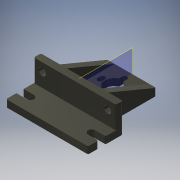
# Autodesk Inventor part: Z Nut Braket 1.0
Saved by Autodesk Inventor 2016 (Build 200138000, 138)
## iProperties
Created: 2017-04-04
Part Number: Z Nut Braket 1.0
Material: PC/ABS Plastic
Document SubType Name: Modeling
Designer: Scott
Density: 0.357273 g/cm^3
Appearance: Gunmetal
Author: Scott
Autodesk Inventor part; units mm, degrees
ref_plane "YZ Plane" through (0, 0, 0) normal (1, 0, 0) x (0, 1, 0)
ref_plane "XZ Plane" through (0, 0, 0) normal (0, 1, 0) x (-1, 0, 0)
sketch "Sketch1" plane through (0, 0, 0) normal (0, 0, 1) x (1, 0, 0)
  line L0 (9.5028, 23.3821) -> (9.5028, -12.6179)
  line L1 (14.5028, 23.3821) -> (14.5028, -12.6179)
  line L2 (26.5028, -12.6179) -> (26.5028, -37.6179)
  line L3 (-32.4972, -17.6179) -> (26.5028, -17.6179)
  line L4 (-32.4972, -12.6179) -> (-20.4972, -12.6179)
  line L5 (-15.4972, -12.6179) -> (9.5028, -12.6179)
  line L6 (14.5028, -12.6179) -> (26.5028, -12.6179)
  line L7 (-20.4972, 23.3821) -> (14.5028, 23.3821)
  line L8 (-15.4972, 23.3821) -> (-15.4972, -12.6179)
  line L9 (-20.4972, 23.3821) -> (-20.4972, -12.6179)
  line L10 (-32.4972, -37.6179) -> (26.5028, -37.6179)
  line L11 (-32.4972, -12.6179) -> (-32.4972, -37.6179)
  line L12 (-2.9972, 1.3821) -> (-2.9972, 17.3821) construction
  line L13 (5.0028, 9.3821) -> (-10.9972, 9.3821) construction
  circle A0 centre (-2.9972, 9.3821) radius 8 construction
  line L14 (-2.9972, 10.3821) -> (-2.9972, 8.3821) construction
  line L15 (-8.4972, 10.3821) -> (-8.4972, 8.3821)
  line L16 (2.5028, 8.3821) -> (2.5028, 10.3821)
  line L17 (-2.9972, 2.3821) -> (-2.9972, 0.3821) construction
  line L18 (-4.7472, 2.3821) -> (-4.7472, 0.3821)
  line L19 (-1.2472, 0.3821) -> (-1.2472, 2.3821)
  arc A1 (-4.7472, 0.3821) -> (-1.2472, 0.3821) centre (-2.9972, 0.3821) ccw
  line L20 (-10.9972, 10.3821) -> (-10.9972, 8.3821) construction
  line L21 (-12.7472, 10.3821) -> (-12.7472, 8.3821)
  line L22 (-9.2472, 8.3821) -> (-9.2472, 10.3821)
  arc A2 (-9.2472, 10.3821) -> (-12.7472, 10.3821) centre (-10.9972, 10.3821) ccw
  arc A3 (-12.7472, 8.3821) -> (-9.2472, 8.3821) centre (-10.9972, 8.3821) ccw
  line L23 (5.0028, 10.3821) -> (5.0028, 8.3821) construction
  line L24 (3.2528, 10.3821) -> (3.2528, 8.3821)
  line L25 (6.7528, 8.3821) -> (6.7528, 10.3821)
  arc A4 (6.7528, 10.3821) -> (3.2528, 10.3821) centre (5.0028, 10.3821) ccw
  arc A5 (3.2528, 8.3821) -> (6.7528, 8.3821) centre (5.0028, 8.3821) ccw
  line L26 (-2.9972, 18.3821) -> (-2.9972, 16.3821) construction
  line L27 (-1.2472, 18.3821) -> (-1.2472, 16.3821)
  line L28 (-4.7472, 16.3821) -> (-4.7472, 18.3821)
  arc A6 (-1.2472, 18.3821) -> (-4.7472, 18.3821) centre (-2.9972, 18.3821) ccw
  arc A7 (-1.2472, 2.3821) -> (-1.4087, 3.1165) centre (-2.9972, 2.3821) ccw
  arc A8 (-4.5856, 3.1165) -> (-4.7472, 2.3821) centre (-2.9972, 2.3821) ccw
  arc A9 (-8.4972, 8.3821) -> (-4.5856, 3.1165) centre (-2.9972, 8.3821) ccw
  arc A10 (-1.4087, 3.1165) -> (2.5028, 8.3821) centre (-2.9972, 8.3821) ccw
  arc A11 (-4.7472, 16.3821) -> (-4.5856, 15.6478) centre (-2.9972, 16.3821) ccw
  arc A12 (-1.4087, 15.6478) -> (-1.2472, 16.3821) centre (-2.9972, 16.3821) ccw
  arc A13 (2.5028, 10.3821) -> (-1.4087, 15.6478) centre (-2.9972, 10.3821) ccw
  arc A14 (-4.5856, 15.6478) -> (-8.4972, 10.3821) centre (-2.9972, 10.3821) ccw
  point P0 (0, 0)
  point P1 (14.5028, 29.202)
  point P2 (-20.4972, 29.202)
  dimension "d51" = 16
  dimension "d52" = 5
  dimension "d53" = 5
  dimension "d54" = 25
  dimension "d55" = 5
  dimension "d56" = 20
  dimension "d58" = 27
  dimension "d59" = 14
  dimension "d60" = 12
  dimension "d61" = 12
  dimension "d64" = 12.5
  dimension "d66" = 2
  dimension "d67" = 3.5
  dimension "d68" = 2
  dimension "d69" = 3.5
  dimension "d70" = 2
  dimension "d71" = 3.5
  dimension "d72" = 2
  dimension "d73" = 3.5
  dimension "d74" = 2
  constraints: 68 end point, 33 point on circle, 22 tangent, 15 centre point, 13 parallel, 8 point on line, 7 midpoint, 5 vertical, 3 coincident, 2 collinear, 2 horizontal
  measures "d51" diameter of A0
  measures "d52" distance between parallel lines of L9 L8
  measures "d53" distance between parallel lines of L1 L0
  measures "d54" distance between parallel lines of L8 L0
  measures "d55" distance between parallel lines of L4 L3
  measures "d56" distance between parallel lines of L10 L3
  measures "d58" distance between parallel lines of L13 L3
  measures "d59" distance between parallel lines of L7 L13
  measures "d60" distance between parallel lines of L1 L2
  measures "d61" distance between parallel lines of L11 L9
  measures "d64" distance between parallel lines of L0 L12
  measures "d66" distance of L15.start L15.end
  measures "d67" diameter of A1
  measures "d68" distance of L18.start L18.end
  measures "d69" diameter of A3
  measures "d70" distance of L21.start L21.end
  measures "d71" diameter of A5
  measures "d72" distance of L25.start L25.end
  measures "d73" distance between parallel lines of L28 L27
  measures "d74" distance of L28.start L28.end
extrude "Extrusion1" add sketch "Sketch1" along normal blind 5
sketch "Sketch2" plane through (0, 0, 5) normal (0, 0, 1) x (1, 0, 0)
  line L0 (26.5028, -37.6179) -> (26.5028, -12.6179) projected
  line L1 (-32.4972, -12.6179) -> (26.5028, -12.6179)
  line L2 (26.5028, -12.6179) -> (26.5028, -17.6179)
  line L3 (26.5028, -17.6179) -> (-32.4972, -17.6179)
  line L4 (-32.4972, -17.6179) -> (-32.4972, -12.6179)
  line L5 (-32.4972, -12.6179) -> (-32.4972, -37.6179) projected
  line L6 (26.5028, -12.6179) -> (14.5028, -12.6179) projected
  point P0 (0, 0)
  dimension "d30" = 5
  constraints: 8 end point, 2 collinear, 2 parallel, 1 horizontal, 1 perpendicular, 1 point on line
  measures "d30" distance between parallel lines of L1 L3
extrude "Extrusion2" add sketch "Sketch2" along normal blind 16
sketch "Sketch3" plane through (14.5028, -12.6179, 0) normal (1, 0, 0) x (0, 0, -1)
  line L0 (0, 0) -> (-21, 0) projected
  line L1 (-5, 0) -> (-5, 36) projected
  line L2 (-21, 0) -> (-5, 0)
  line L3 (-5, 36) -> (-20, 0)
  point P0 (0, 12.6179)
  point P1 (-5, 31)
  dimension "d77" = 15
  constraints: 4 end point, 1 perpendicular, 1 point on line
  measures "d77" distance from line of L1 L3.end
extrude "Extrusion3" add sketch "Sketch3" against normal blind 5
sketch "Sketch4" plane through (14.5028, -12.6179, 0) normal (0, 1, 0) x (1, 0, 0)
  circle A0 centre (6, -15) radius 2.6
  line L0 (12, 0) -> (12, -21) projected
  line L1 (12, -21) -> (-47, -21) projected
  point P0 (-14.5028, 0)
  point P1 (0, -25)
  dimension "d36" = 5.2
  dimension "d37" = 6
  dimension "d38" = 6
  constraints: 1 centre point, 1 other
  measures "d36" diameter of A0
  measures "d37" distance from line of L0 A0.centre
extrude "Extrusion4" cut sketch "Sketch4" against normal through all
sketch "Sketch5" plane through (0, 0, 5) normal (0, 0, 1) x (1, 0, 0)
  arc A0 (19.0028, -25.0179) -> (19.0028, -30.2179) centre (19.0028, -27.6179) ccw
  line L0 (26.5028, -37.6179) -> (26.5028, -17.6179) projected
  line L1 (-32.4972, -37.6179) -> (26.5028, -37.6179) projected
  line L2 (19.0028, -25.0179) -> (26.5028, -25.0179)
  line L3 (19.0028, -30.2179) -> (26.5028, -30.2179)
  line L4 (26.5028, -37.6179) -> (26.5028, -12.6179) projected
  line L5 (26.5028, -25.0179) -> (26.5028, -30.2179)
  point P0 (0, 0)
  point P1 (-34.4972, -33.6179)
  point P2 (17.5028, -33.6179)
  dimension "d41" = 7.5
  dimension "d42" = 10
  dimension "d43" = 5.2
  constraints: 6 end point, 2 point on circle, 2 point on line, 2 tangent, 1 centre point, 1 collinear, 1 horizontal, 1 perpendicular, 1 other
  measures "d41" distance from line of L0 A0.centre
  measures "d43" diameter of A0
extrude "Extrusion5" cut sketch "Sketch5" against normal blind 5
fillet "Fillet1" radius 1 5 edges at (-32.4972, -12.6179, 10.5) (-32.4972, -17.6179, 13) (26.5028, -30.2179, 2.5) (26.5028, -25.0179, 2.5) (26.5028, -17.6179, 13)
ref_plane "Work Plane2" through (-2.9972, 0.3821, 0) normal (1, 0, 0) x (0, 0, 1)
mirror "Mirror2" about plane through (-2.9972, 0.3821, 0) normal (1, 0, 0) of "Extrusion5", "Extrusion4", "Extrusion3"
fillet "Fillet2" radius 1 8 edges at (14.5028, 23.3821, 2.5) (-20.4972, 23.3821, 2.5) (26.5028, -37.6179, 2.5) (-32.4972, -37.6179, 2.5) (-1.4087, 3.1165, 2.5) (-4.5856, 3.1165, 2.5) (-1.4087, 15.6478, 2.5) (-4.5856, 15.6478, 2.5)
ref_plane "Work Plane3" through (-2.9972, -12.6179, 0) normal (-1, 0, 0) x (0, 0, 1)
body "Solid1"
